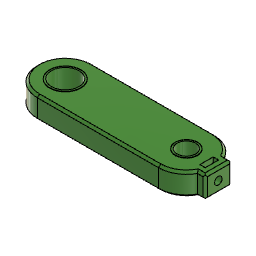
Picavet_entraxe v4 (Autodesk Fusion 360 design; units mm, degrees)
Autodesk Fusion 360 part; units mm, degrees
sketch "Esquisse1" plane through (0, 0, 0) normal (0, 0, 1) x (1, 0, 0)
  circle A0 centre (-55.5807, 0.978) radius 6.2
  circle A1 centre (-1.1807, 0.978) radius 4.2
  line L0 (-55.5807, 13.478) -> (-1.1807, 13.478)
  line L1 (-1.1807, 13.478) -> (-1.1807, -11.522) construction
  line L2 (-1.1807, -11.522) -> (-55.5807, -11.522)
  line L3 (-55.5807, -11.522) -> (-55.5807, 13.478) construction
  arc A2 (-55.5807, 13.478) -> (-55.5807, -11.522) centre (-55.5807, 0.978) ccw
  line L4 (9.7852, -5.022) -> (13.2852, -5.022)
  line L5 (13.2852, -5.022) -> (13.2852, 6.978)
  line L6 (13.2852, 6.978) -> (9.7852, 6.978)
  arc A3 (-1.1807, -11.522) -> (9.7852, -5.022) centre (-1.1807, 0.978) ccw
  arc A4 (9.7852, 6.978) -> (-1.1807, 13.478) centre (-1.1807, 0.978) ccw
  dimension "d1" = 54.4
  dimension "d2" = 12.4
  dimension "d3" = 8.4
  dimension "d4" = 25
  dimension "d5" = 12.5
  dimension "d7" = 12
  dimension "d8" = 3.5
  constraint horizontal L0
  constraint vertical L1
  constraint horizontal L2
  constraint vertical L3
  constraint coincident A0.centre L3
  constraint coincident A1.centre L1
  constraint coincident A0.centre A2.centre
  constraint coincident A1.centre A3.centre
  constraint horizontal L4
  constraint vertical L5
  constraint horizontal L6
  constraint coincident L6.end A3
  constraint concentric A3 A4
  measures "d1" distance of A0.centre A1.centre
  measures "d2" diameter of A0
  measures "d3" diameter of A1
  measures "d4" distance of L0.start L2.end
  measures "d5" distance of A0.centre L2
  measures "d7" distance of L4.start L6.end
  measures "d8" distance of L4.start L4.end
extrude "Extrusion1" add sketch "Esquisse1" along normal blind 10
sketch "Esquisse2" plane through (0, 0, 10) normal (0, 0, 1) x (-1, 0, 0)
  circle A0 centre (55.5807, -0.978) radius 6.2
  circle A1 centre (1.1807, -0.978) radius 4.2
  arc A2 (1.1807, 11.522) -> (-9.7852, 5.022) centre (1.1807, -0.978) ccw
  line L0 (-9.7852, 5.022) -> (-13.2852, 5.022)
  line L1 (-13.2852, 5.022) -> (-13.2852, -6.978)
  line L2 (-13.2852, -6.978) -> (-9.7852, -6.978)
  arc A3 (-9.7852, -6.978) -> (1.1807, -13.478) centre (1.1807, -0.978) ccw
  line L3 (1.1807, -13.478) -> (55.5807, -13.478)
  arc A4 (55.5807, -13.478) -> (55.5807, 11.522) centre (55.5807, -0.978) ccw
  line L4 (55.5807, 11.522) -> (1.1807, 11.522)
  circle A5 centre (55.5807, -0.978) radius 7
  circle A6 centre (1.1807, -0.978) radius 5
  dimension "d11" = 14
  dimension "d12" = 10
  constraint concentric A0 A5
  constraint concentric A1 A6
  measures "d11" diameter of A5
  measures "d12" diameter of A6
extrude "Extrusion2" add sketch "Esquisse2" along normal blind 0.2 contours A5 | A6
ref_plane "Plan de construction2" through (10.2852, 0.978, 5) normal (1, 0, 0) x (0, 1, 0)
sketch "Esquisse3" plane through (10.2852, 0, 0) normal (1, 0, 0) x (0, 1, 0)
  line L0 (-5.022, 0) -> (6.978, 0)
  line L1 (6.978, 0) -> (6.978, 10)
  line L2 (6.978, 10) -> (-5.022, 10)
  line L3 (-5.022, 10) -> (-5.022, 0)
  line L4 (-2.022, 10) -> (3.978, 10)
  line L5 (3.978, 10) -> (3.978, 5)
  line L6 (3.978, 5) -> (-2.022, 5) construction
  line L7 (-2.022, 5) -> (-2.022, 10)
  line L8 (0.978, 5) -> (0.978, 1.9) construction
  line L9 (-2.022, 6.7321) -> (-2.022, 3.2679)
  line L10 (-2.022, 3.2679) -> (0.978, 1.5359)
  line L11 (0.978, 1.5359) -> (3.978, 3.2679)
  line L12 (3.978, 3.2679) -> (3.978, 6.7321)
  point P0 (0.978, 5)
  dimension "d15" = 3.1
  dimension "d16" = 5
  dimension "d17" = 6
  dimension "d18" = 12
  dimension "d19" = 3
  constraint horizontal L4
  constraint vertical L5
  constraint horizontal L6
  constraint vertical L7
  constraint midpoint L6 P0
  constraint perpendicular L6 L8
  constraint coincident P0 L8.start
  measures "d15" distance of P0 L8.end
  measures "d16" distance of L4.end L5.end
  measures "d17" distance of L4.start L4.end
  measures "d18" distance of L0.start L0.end
  measures "d19" distance of L3 L7
extrude "Extrusion3" cut sketch "Esquisse3" against normal blind 2.4 contours L2 L4 L5 L7 L9 L10 L11 L12
hole "Perçage1" at (13.2852, 0.8569, 5) direction (-1, 0, 0) diameter 3.4 depth 11 tip angle 180
chamfer "Chanfrein1" distance 1 angle 45 16 edges at (5.1931, -9.7749, 10) (5.1931, 11.7309, 10) (-28.3807, 13.478, 10) (-68.0807, 0.978, 10) (-28.3807, -11.522, 10) (-28.3807, -11.522, 0) (-68.0807, 0.978, 0) (-28.3807, 13.478, 0) (5.1931, 11.7309, 0) (5.1931, -9.7749, 0) (11.5352, -5.022, 0) (11.5352, -5.022, 10) (13.2852, 0.978, 0) (13.2852, 0.978, 10) (11.5352, 6.978, 10) (11.5352, 6.978, 0)
chamfer "Chanfrein2" distance 1 angle 45 2 edges at (13.2852, 6.978, 5) (13.2852, -5.022, 5)
equation "d5 = d4 / 2"
equation "d19 = ( d18 - d17 ) / 2"
